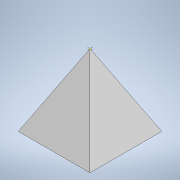
# Autodesk Inventor part: HexSideSpike
Saved by Autodesk Inventor 2020 (Build 240168000, 168)
## iProperties
Created: 2023-12-28
Part Number: HexSideSpike
Material: Generic
Document SubType Name: Modeling
Designer: smz3rm
Density: 1 g/cm^3
Appearance: Default
Author: smz3rm
Autodesk Inventor part; units mm, degrees
ref_plane "YZ Plane" through (0, 0, 0) normal (1, 0, 0) x (0, 1, 0)
ref_plane "XZ Plane" through (0, 0, 0) normal (0, 1, 0) x (-1, 0, 0)
ref_plane "XY Plane" through (0, 0, 0) normal (0, 0, 1) x (1, 0, 0)
sketch "Sketch1" plane through (0, 0, 0) normal (0, 1, 0) x (-1, 0, 0)
  line L0 (7.5, 7.5) -> (-7.5, 7.5)
  line L1 (-7.5, 7.5) -> (-7.5, -7.5)
  line L2 (-7.5, -7.5) -> (7.5, -7.5)
  line L3 (7.5, -7.5) -> (7.5, 7.5)
  line L4 (7.5, 7.5) -> (-7.5, -7.5) construction
  line L5 (-7.5, 7.5) -> (7.5, -7.5) construction
  point P0 (0, 0)
  dimension "d0" = 15
  dimension "d1" = 15
  constraints: 12 end point, 2 midpoint, 2 parallel, 1 horizontal, 1 perpendicular
  measures "d0" distance of L2.end L1.end
  measures "d1" distance of L1.end L0.end
extrude "Extrusion1" add sketch "Sketch1" along normal blind 15
sketch "Sketch2" plane through (0, 15, 0) normal (0, 1, 0) x (1, 0, 0)
  point P0 (0, 0)
  point P1 (0, 0)
  constraints: 1 coincident
ref_plane "Work Plane1" through (7.5, 0, 7.5) normal (0.8944272, 0.4472136, 0) x (0, 0, -1)
ref_plane "Work Plane2" through (-7.5, 0, 7.5) normal (0, 0.4472136, 0.8944272) x (1, 0, 0)
ref_plane "Work Plane3" through (-7.5, 0, -7.5) normal (0.8944272, -0.4472136, 0) x (0.4082483, 0.8164966, 0.4082483)
ref_plane "Work Plane4" through (7.5, 0, -7.5) normal (0, 0.4472136, -0.8944272) x (-1, 0, 0)
sketch "Sketch4" plane through (7.5, 0, 7.5) normal (0.8944272, 0.4472136, 0) x (0, 0, -1)
  line L0 (26.6476, 25.9998) -> (-15.2684, 25.9998)
  line L1 (-15.2684, 25.9998) -> (-15.2684, -13.1545)
  line L2 (-15.2684, -13.1545) -> (26.6476, -13.1545)
  line L3 (26.6476, -13.1545) -> (26.6476, 25.9998)
  point P0 (7.5, 3.3541)
  constraints: 8 end point, 2 parallel, 1 horizontal, 1 perpendicular
extrude "Extrusion2" cut sketch "Sketch4" along normal through all
sketch "Sketch5" plane through (-7.5, 0, 7.5) normal (0, 0.4472136, 0.8944272) x (1, 0, 0)
  line L0 (25.5392, 33.5657) -> (-14.5967, 33.5657)
  line L1 (-14.5967, 33.5657) -> (-14.5967, -23.0742)
  line L2 (-14.5967, -23.0742) -> (25.5392, -23.0742)
  line L3 (25.5392, -23.0742) -> (25.5392, 33.5657)
  point P0 (7.5, 3.3541)
  constraints: 8 end point, 2 parallel, 1 horizontal, 1 perpendicular
extrude "Extrusion3" cut sketch "Sketch5" along normal through all
sketch "Sketch6" plane through (-7.5, 0, -7.5) normal (0.8944272, -0.4472136, 0) x (0.4082483, 0.8164966, 0.4082483)
  line L0 (35.4927, -22.9081) -> (-17.0623, -22.9081)
  line L1 (-17.0623, -22.9081) -> (-17.0623, 39.3429)
  line L2 (-17.0623, 39.3429) -> (35.4927, 39.3429)
  line L3 (35.4927, 39.3429) -> (35.4927, -22.9081)
  point P0 (6.1237, 5.4772)
  constraints: 8 end point, 2 parallel, 1 horizontal, 1 perpendicular
extrude "Extrusion4" cut sketch "Sketch6" against normal blind 15
sketch "Sketch7" plane through (7.5, 0, -7.5) normal (0, 0.4472136, -0.8944272) x (-1, 0, 0)
  line L0 (-15.9671, 26.9617) -> (32.6533, 26.9617)
  line L1 (32.6533, 26.9617) -> (32.6533, -21.7992)
  line L2 (32.6533, -21.7992) -> (-15.9671, -21.7992)
  line L3 (-15.9671, -21.7992) -> (-15.9671, 26.9617)
  point P0 (7.5, 3.3541)
  constraints: 8 end point, 2 parallel, 1 horizontal, 1 perpendicular
extrude "Extrusion5" cut sketch "Sketch7" along normal through all
equation "\"d0\" = 0.5 * BodyHeight"
equation "\"d1\" = 0.5 * BodyHeight"
equation "\"d2\" = 0.5 * BodyHeight"
equation "\"d8\" = 0.5 * BodyHeight"
equation "\"BodyHeight\" = 30"
body "Solid1"
